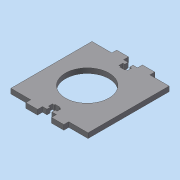
# Autodesk Inventor part: Part3
Saved by Autodesk Inventor 2016 SP1 (Build 200210100, 210)
## iProperties
Created: 2016-03-20
Part Number: Part3
Material: Generic
Document SubType Name: Modeling
Designer: Mohamed A.
Density: 1 g/cm^3
Appearance: Default
Author: Mohamed A.
Autodesk Inventor part; units mm, degrees
ref_plane "YZ Plane" through (0, 0, 0) normal (1, 0, 0) x (0, 1, 0)
ref_plane "XZ Plane" through (0, 0, 0) normal (0, 1, 0) x (-1, 0, 0)
ref_plane "XY Plane" through (0, 0, 0) normal (0, 0, 1) x (1, 0, 0)
sketch "Sketch1" plane through (0, 0, 0) normal (0, 0, 1) x (1, 0, 0)
  circle A0 centre (-1.6325, 0) radius 5.15 construction
  circle A1 centre (-1.6325, 0) radius 13.25 projected
  line L0 (10.9595, -23.5) -> (10.9595, 23.5) construction
  line L1 (-21.7072, 23.5) -> (-21.7072, -23.5) construction
  line L2 (11.8175, -24.7) -> (11.8175, -27.7)
  line L3 (11.8175, -27.7) -> (4.3175, -27.7)
  circle A2 centre (-1.6325, 0) radius 13.25 construction
  line L4 (-5.8325, -4.2) -> (-5.8325, 4.2) construction
  line L5 (-5.8325, 4.2) -> (12.0675, 4.2) construction
  line L6 (12.0675, 4.2) -> (12.0675, -4.2) construction
  line L7 (12.0675, -4.2) -> (-5.8325, -4.2) construction
  circle A3 centre (-17.9325, 18) radius 2.75 construction
  circle A4 centre (18.0675, 18) radius 2.75 construction
  circle A5 centre (-17.9325, -18) radius 2.75 construction
  circle A6 centre (18.0675, -18) radius 2.75 construction
  circle A7 centre (10.0175, 10.5) radius 2 construction
  circle A8 centre (-2.4825, 10.5) radius 2 construction
  circle A9 centre (-2.4825, -10.5) radius 2 construction
  circle A10 centre (10.0175, -10.5) radius 2 construction
  line L8 (-23.4325, 23.5) -> (-23.4325, -23.5) construction
  line L9 (23.5675, -23.5) -> (23.5675, 23.5) construction
  line L10 (23.5675, 23.5) -> (-23.4325, 23.5) construction
  line L11 (4.3175, -27.7) -> (4.3175, -24.7)
  line L12 (1.5675, -24.7) -> (1.5675, -22.7)
  line L13 (1.5675, -22.7) -> (2.7175, -22.7)
  line L14 (2.7175, -20.3) -> (2.7175, -22.7)
  line L15 (2.7175, -20.3) -> (1.5675, -20.3)
  line L16 (1.5675, -20.3) -> (1.5675, -19.7)
  line L17 (1.5675, -19.7) -> (-1.4325, -19.7)
  line L18 (-1.4325, -19.7) -> (-1.4325, -20.3)
  line L19 (-1.4325, -20.3) -> (-2.5825, -20.3)
  line L20 (-2.5825, -20.3) -> (-2.5825, -22.7)
  line L21 (-2.5825, -22.7) -> (-1.4325, -22.7)
  line L22 (-1.4325, -24.7) -> (-1.4325, -22.7)
  line L23 (-4.1825, -24.7) -> (-4.1825, -27.7)
  line L24 (0.0675, -17.369) -> (0.0675, -28.5133) construction
  line L25 (-4.1825, -27.7) -> (-11.3405, -27.7)
  line L26 (4.3175, -27.7) -> (-4.1825, -27.7) construction
  line L27 (1.5675, -24.7) -> (4.3175, -24.7)
  line L28 (-1.4325, -24.7) -> (-4.1825, -24.7)
  line L29 (-4.1825, -24.7) -> (-1.4325, -24.7)
  line L30 (-32.8325, 0) -> (32.9675, 0) construction
  line L31 (11.8175, -24.7) -> (23.5675, -24.7)
  line L32 (1.5675, -24.7) -> (4.3175, -24.7)
  line L33 (-11.3405, -27.7) -> (-11.3405, -24.7)
  line L34 (-11.3405, -24.7) -> (-23.4325, -24.7)
  line L35 (-23.4325, -24.7) -> (-23.4325, -23.5)
  line L36 (23.5675, -24.7) -> (23.5675, -23.5)
  line L37 (10.9595, 23.5) -> (10.9595, -23.5) construction
  line L38 (-21.7072, -23.5) -> (-21.7072, 23.5) construction
  line L39 (11.8175, 24.7) -> (11.8175, 27.7)
  line L40 (11.8175, 27.7) -> (4.3175, 27.7)
  circle A11 centre (-17.9325, 18) radius 2.75 construction
  circle A12 centre (18.0675, 18) radius 2.75 construction
  line L41 (4.3175, 27.7) -> (4.3175, 24.7)
  line L42 (1.5675, 24.7) -> (1.5675, 22.7)
  line L43 (1.5675, 22.7) -> (2.7175, 22.7)
  line L44 (2.7175, 20.3) -> (2.7175, 22.7)
  line L45 (2.7175, 20.3) -> (1.5675, 20.3)
  line L46 (1.5675, 20.3) -> (1.5675, 19.7)
  line L47 (1.5675, 19.7) -> (-1.4325, 19.7)
  line L48 (-1.4325, 19.7) -> (-1.4325, 20.3)
  line L49 (-1.4325, 20.3) -> (-2.5825, 20.3)
  line L50 (-2.5825, 20.3) -> (-2.5825, 22.7)
  line L51 (-2.5825, 22.7) -> (-1.4325, 22.7)
  line L52 (-1.4325, 24.7) -> (-1.4325, 22.7)
  line L53 (-4.1825, 24.7) -> (-4.1825, 27.7)
  line L54 (0.0675, 17.369) -> (0.0675, 28.5133) construction
  line L55 (-4.1825, 27.7) -> (-11.3405, 27.7)
  line L56 (4.3175, 27.7) -> (-4.1825, 27.7) construction
  line L57 (1.5675, 24.7) -> (4.3175, 24.7)
  line L58 (-1.4325, 24.7) -> (-4.1825, 24.7)
  line L59 (-4.1825, 24.7) -> (-1.4325, 24.7)
  line L60 (11.8175, 24.7) -> (23.5675, 24.7)
  line L61 (1.5675, 24.7) -> (4.3175, 24.7)
  line L62 (-11.3405, 27.7) -> (-11.3405, 24.7)
  line L63 (-11.3405, 24.7) -> (-23.4325, 24.7)
  line L64 (-23.4325, 24.7) -> (-23.4325, 23.5)
  line L65 (23.5675, 24.7) -> (23.5675, 23.5)
  line L66 (23.5675, 23.5) -> (23.5675, -23.5)
  line L67 (-23.4325, -23.5) -> (-23.4325, 23.5)
  point P0 (0, 0)
  dimension "d11" = 47
  dimension "d12" = 11.75
  dimension "d18" = 3
  dimension "d19" = 5.3
  dimension "d20" = 2.4
  dimension "d21" = 5
  dimension "d22" = 8
  dimension "d23" = 7.5
  dimension "d24" = 3
  dimension "d25" = 4.2
  dimension "d26" = 8.5
  dimension "d27" = 23.158
  constraints: 112 end point, 32 symmetric about line, 23 perpendicular, 18 point on line, 9 collinear, 4 vertical, 5 other
  measures "d11" distance between parallel lines of L8 L9
  measures "d12" distance between parallel lines of L2 L9
  measures "d18" distance between parallel lines of L22 L12
  measures "d19" distance between parallel lines of L20 L14
  measures "d20" distance between parallel lines of L13 L15
  measures "d21" distance between parallel lines of L3 L13
  measures "d22" distance between parallel lines of L3 L17
  measures "d23" distance between parallel lines of L11 L2
  measures "d24" distance between parallel lines of L31 L3
  measures "d25" distance from line of L8.end L25
  measures "d26" distance between parallel lines of L23 L11
  measures "d27" distance between parallel lines of L33 L2
extrude "Extrusion1" add sketch "Sketch1" along normal blind 3
equation "\"d12\" = 0.25 * d11"
body "Solid1"
